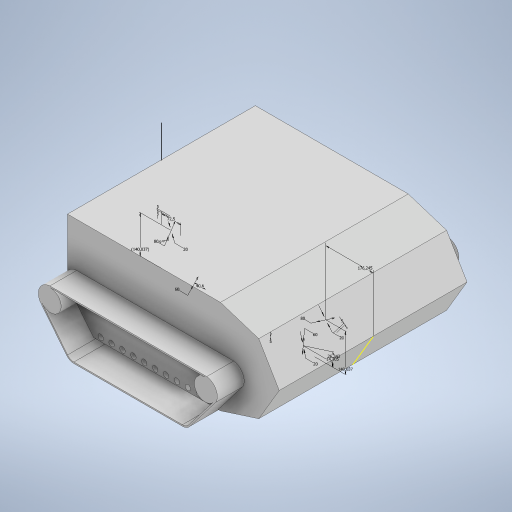
# Autodesk Inventor part: 03-10-2023 proget work
Saved by Autodesk Inventor 2023 (Build 270158000, 158)
## iProperties
Created: 2023-03-10
Part Number: 03-10-2023 proget work
Material: Generico
Document SubType Name: Modeling
Designer: Admin
Density: 1 g/cm^3
Appearance: Default
Author: Admin
Autodesk Inventor part; units mm, degrees
ref_plane "YZ Plane" through (0, 0, 0) normal (1, 0, 0) x (0, 1, 0)
ref_plane "XZ Plane" through (0, 0, 0) normal (0, 1, 0) x (-1, 0, 0)
ref_plane "XY Plane" through (0, 0, 0) normal (0, 0, 1) x (1, 0, 0)
sketch "Schizzo1" plane through (0, 0, 0) normal (0, 0, 1) x (1, 0, 0)
  line L0 (0, 0) -> (600, 0)
  line L1 (600, 0) -> (600, 350) construction
  line L2 (600, 350) -> (0, 350)
  line L3 (0, 350) -> (0, 0)
  line L4 (600, 350) -> (742.8332, 304.1887)
  line L5 (600, 350) -> (750, 350) construction
  line L6 (742.8332, 304.1887) -> (819.0584, 175)
  line L7 (819.0584, 175) -> (742.8332, 45.8113)
  line L8 (742.8332, 45.8113) -> (600, 0)
  line L9 (0, 0) -> (30, 0)
  line L10 (30, 0) -> (30, 30)
  line L11 (30, 30) -> (600, 30)
  line L12 (30, 350) -> (30, 320)
  line L13 (30, 320) -> (30, 30)
  line L14 (30, 320) -> (600, 320)
  line L15 (600, 320) -> (724.9503, 279.9243)
  line L16 (724.9503, 279.9243) -> (788.2304, 172.6755)
  line L17 (788.2304, 172.6755) -> (728.3337, 71.1608)
  line L18 (600, 30) -> (728.3337, 71.1608)
  dimension "d0" = 600
  dimension "d1" = 350
  dimension "d3" = 150
  dimension "d6" = 150
  dimension "d7" = 150
  dimension "d8" = 150
  dimension "d9" = 17.783
  dimension "d10" = 59.458
  dimension "d11" = 30
  dimension "d12" = 30
  dimension "d13" = 30
  dimension "d15" = 117.8679
  dimension "d16" = 124.5258
  constraints: 38 end point, 6 parallel, 5 perpendicular, 4 point on line, 2 horizontal, 1 vertical
  measures "d0" distance of L2.end L1.end
  measures "d1" distance of L1.end L0.end
  measures "d3" distance of L1.end L4.end
  measures "d6" distance of L4.end L6.end
  measures "d7" distance of L6.end L7.end
  measures "d8" distance of L7.end L0.end
  measures "d9" angle of L5 L4
  measures "d10" angle of L5 L6
  measures "d11" distance of L0.start L9.end
  measures "d12" distance of L9.end L10.end
  measures "d13" distance of L12.start L12.end
  measures "d15" distance of L16.end L17.end
  measures "d16" distance of L15.end L16.end
extrude "Estrusione1" add sketch "Schizzo1" along normal mid plane 700 contours L10 L11 L18 L17 L16 L15 L14 L12 L2 L4 L6 L7 L8 L0 | L13 L14 L15 L16 L17 L18 L11
extrude "Estrusione2" cut sketch "Schizzo1" along normal mid plane 600 contours L13 L14 L15 L16 L17 L18 L11
sketch "Schizzo2" plane through (0, 0, 0) normal (0, 0, 1) x (1, 0, 0)
  line L0 (30, 0) -> (30, 350) projected
  line L1 (600, 30) -> (30, 30) projected
  line L2 (30, 470.1492) -> (30, 30)
  line L3 (819.0584, 175) -> (742.8332, 45.8113) projected
  line L4 (30, 250.0746) -> (30, 30)
  line L5 (30, 140.0373) -> (102.5, 140.0373)
  circle A0 centre (66.25, 140.0373) radius 10
  circle A1 centre (642.8131, 140.0373) radius 10
  line L6 (66.25, 140.0373) -> (179.04, 140.0373) construction
  circle A2 centre (153.7896, 14.3054) radius 10
  circle A3 centre (558.3484, 14.3054) radius 10
  circle A4 centre (194.3896, 14.3054) radius 10
  circle A5 centre (234.9896, 14.3054) radius 10
  circle A6 centre (275.5896, 14.3054) radius 10
  circle A7 centre (316.1896, 14.3054) radius 10
  circle A8 centre (356.7896, 14.3054) radius 10
  circle A9 centre (397.3896, 14.3054) radius 10
  circle A10 centre (437.9896, 14.3054) radius 10
  circle A11 centre (478.5896, 14.3054) radius 10
  circle A12 centre (519.1896, 14.3054) radius 10
  line L7 (66.25, 140.0373) -> (153.7896, 14.3054) construction
  line L8 (153.7896, 14.3054) -> (558.3484, 14.3054) construction
  circle A13 centre (642.8131, 140.0373) radius 40
  circle A14 centre (66.25, 140.0373) radius 40
  line L9 (66.25, 140.0373) -> (638.5139, 140.0373) construction
  line L10 (65.8113, 180.0349) -> (642.3744, 180.0349)
  circle A15 centre (558.3484, 14.3054) radius 30
  circle A16 centre (153.7896, 14.3054) radius 30
  line L11 (671.2763, 111.9332) -> (582.1291, -3.9835)
  line L12 (558.3484, -15.6946) -> (153.7896, -15.6946)
  line L13 (130.3406, -4.4068) -> (34.9847, 115.0878)
  line L14 (64.1021, 185.0349) -> (648.9858, 185.0349)
  line L15 (683.165, 119.1901) -> (586.0925, -7.0316)
  line L16 (558.3484, -20.6946) -> (153.7896, -20.6946)
  line L17 (126.4324, -7.5255) -> (29.7686, 113.6081)
  arc A17 (126.4324, -7.5255) -> (153.7896, -20.6946) centre (153.7896, 14.3054) ccw
  arc A18 (64.1021, 185.0349) -> (29.7686, 113.6081) centre (66.25, 140.0373) ccw
  line L18 (30, 0) -> (600, 0) projected
  arc A19 (683.165, 119.1901) -> (648.9858, 185.0349) centre (642.8131, 140.0373) ccw
  line L19 (600, 0) -> (742.8332, 45.8113) projected
  arc A20 (558.3484, -20.6946) -> (586.0925, -7.0316) centre (558.3484, 14.3054) ccw
  point P0 (0, 0)
  point P1 (120.4271, 0)
  point P2 (126.824, 0)
  point P3 (66.6887, 180.0349)
  point P4 (585.1926, 0)
  point P5 (591.5003, 0)
  dimension "d21" = 72.5
  dimension "d22" = 20
  dimension "d23" = 20
  dimension "d30" = 20
  dimension "d34" = 40.6
  dimension "d41" = 80
  dimension "d42" = 80
  dimension "d73" = 60
  dimension "d74" = 60
  dimension "d78" = 5
  dimension "d80" = 5
  dimension "d81" = 5
  dimension "d83" = 5
  dimension "d84" = 140.0373
  dimension "d85" = 140.0373
  dimension "d86" = 176.2454
  dimension "d87" = 14.3054
  dimension "d88" = 26.3426
  constraints: 31 end point, 21 centre point, 17 point on circle, 8 coincident, 7 horizontal, 6 tangent, 3 midpoint, 2 perpendicular, 2 point on line, 1 parallel, 1 vertical, 18 other
  measures "d21" distance of L5.start L5.end
  measures "d22" diameter of A0
  measures "d23" diameter of A1
  measures "d30" diameter of A3
  measures "d34" distance of L7.end A4.centre
  measures "d41" diameter of A13
  measures "d42" diameter of A14
  measures "d73" diameter of A15
  measures "d74" diameter of A16
  measures "d78" distance between parallel lines of L10 L14
  measures "d80" distance between parallel lines of L12 L16
  measures "d81" distance between parallel lines of L17 L13
  measures "d83" distance between parallel lines of L11 L15
  measures "d84" distance from line of L18 A1.centre
  measures "d85" distance from line of L18 L6.start
  measures "d86" horizontal distance of L3.start A1.centre
  measures "d87" distance from line of L18 L8.end
  measures "d88" distance from line of L19 A15.centre
extrude "Estrusione3" cut sketch "Schizzo2" along normal mid plane 700 contours A15 A12 | A12 A15 | A0 L5 | L5 A0 | A1 | A2 | A3 | A4 | A5 | A6 | A7 | A8 | A9 | A10 | A11
extrude "Estrusione6" add sketch "Schizzo2" along normal mid plane 900 contours A14 L0 | L0 A14
extrude "Estrusione7" cut sketch "Schizzo2" along normal mid plane 750 contours A14 L0 | L0 A14
extrude "Estrusione8" add sketch "Schizzo2" along normal mid plane 700 contours A14 L0 | L0 A14
extrude "Estrusione9" cut sketch "Schizzo2" along normal mid plane 600 contours A14 L0 | L0 A14
extrude "Estrusione10" add sketch "Schizzo2" along normal mid plane 900 contours A13
extrude "Estrusione11" cut sketch "Schizzo2" along normal mid plane 750 contours A13
extrude "Estrusione12" add sketch "Schizzo2" along normal mid plane 700 contours A13
extrude "Estrusione13" cut sketch "Schizzo2" along normal mid plane 600 contours A13
extrude "Estrusione14" add sketch "Schizzo2" along normal mid plane 900 contours A0 L5 | L5 A0 | A1
extrude "Estrusione15" cut sketch "Schizzo2" along normal mid plane 550 contours A0 L5 | L5 A0 | A1
extrude "Estrusione17" add sketch "Schizzo2" along normal mid plane 900 contours L18 L13 A16 L12 A15 L11 L15 A20 L16 A17 L17 | L17 L1 L13 L18 | L17 A18 L0 A14 | L0 A14 L13 L1 L17 | L0 A18 L14 A19 L15 L18 L11 A13 L10 A14
